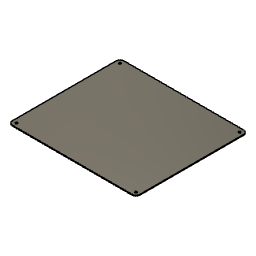
magnetic base plate optics v3 (Autodesk Fusion 360 design; units mm, degrees)
Autodesk Fusion 360 part; units mm, degrees
note: some values were not read from the file. Set by a fixed rule: the direction of a hole.
sketch "Sketch1" plane through (0, 0, 0) normal (0, 1, 0) x (1, 0, 0)
  line L0 (0, 0) -> (400, 0)
  line L1 (400, 0) -> (400, -350)
  line L2 (400, -350) -> (0, -350)
  line L3 (0, -350) -> (0, 0)
  line L4 (12.5, -12.5) -> (387.5, -12.5) construction
  line L5 (387.5, -12.5) -> (387.5, -337.5) construction
  line L6 (387.5, -337.5) -> (12.5, -337.5) construction
  line L7 (12.5, -337.5) -> (12.5, -12.5) construction
  line L8 (0, -175) -> (400, -175) construction
  line L9 (200, 0) -> (200, -350) construction
  dimension "d1" = 350
  dimension "d2" = 400
  dimension "d3" = 325
  dimension "d4" = 375
  constraint horizontal L0
  constraint vertical L1
  constraint horizontal L2
  constraint vertical L3
  constraint coincident L0.start L3.end
  constraint horizontal L4
  constraint vertical L5
  constraint horizontal L6
  constraint vertical L7
  constraint midpoint L3 L8.start
  constraint midpoint L1 L8.end
  constraint midpoint L0 L9.start
  constraint midpoint L2 L9.end
  constraint symmetric L4 L6 L8
  constraint symmetric L5 L7 L9
  measures "d1" distance of L0.start L2.end
  measures "d2" distance of L0.start L0.end
  measures "d3" distance of L4.start L6.end
  measures "d4" distance of L5.end L6.end
extrude "Extrude1" add sketch "Sketch1" along normal blind 2
hole "Hole1" at (12.5, 0, 337.5) at (387.5, 0, 337.5) at (12.5, 0, 12.5) at (387.5, 0, 12.5) direction (0, 1, 0) diameter 6.6 end through all
fillet "Fillet1" radius 12.5 4 edges at (0, 1, 350) (400, 1, 350) (400, 1, 0) (0, 1, 0)
sketch "Sketch2" plane through (0, 0, 0) normal (0, -1, 0) x (1, 0, 0)
  arc A0 (0, 12.5) -> (12.5, 0) centre (12.5, 12.5) ccw
  line L0 (12.5, 0) -> (387.5, 0)
  arc A1 (387.5, 0) -> (400, 12.5) centre (387.5, 12.5) ccw
  line L1 (400, 12.5) -> (400, 337.5)
  arc A2 (400, 337.5) -> (387.5, 350) centre (387.5, 337.5) ccw
  line L2 (387.5, 350) -> (12.5, 350)
  arc A3 (12.5, 350) -> (0, 337.5) centre (12.5, 337.5) ccw
  line L3 (0, 337.5) -> (0, 12.5)
  circle A4 centre (12.5, 12.5) radius 3.3
  circle A5 centre (12.5, 337.5) radius 3.3
  circle A6 centre (387.5, 337.5) radius 3.3
  circle A7 centre (387.5, 12.5) radius 3.3
